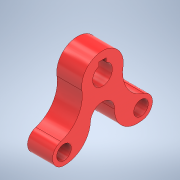
# Autodesk Inventor part: hw5
Saved by Autodesk Inventor 2021 (Build 250183000, 183)
## iProperties
Created: 2022-04-30
Part Number: hw5
Material: Generic
Document SubType Name: Modeling
Designer: authe
Density: 1 g/cm^3
Appearance: Light Red
Author: authe
Autodesk Inventor part; units mm, degrees
ref_plane "YZ Plane" through (0, 0, 0) normal (1, 0, 0) x (0, 1, 0)
ref_plane "XZ Plane" through (0, 0, 0) normal (0, 1, 0) x (-1, 0, 0)
ref_plane "XY Plane" through (0, 0, 0) normal (0, 0, 1) x (1, 0, 0)
sketch "Sketch1" plane through (0, 0, 0) normal (1, 0, 0) x (0, 1, 0)
  point P0 (0, 0)
sketch "Sketch2" plane through (0, 0, 0) normal (1, 0, 0) x (0, 1, 0)
  point P0 (0, 0)
sketch "Sketch3" plane through (0, 0, 0) normal (1, 0, 0) x (0, 1, 0)
  arc A0 (44.1588, 17.5) -> (44.1588, -17.5) centre (0, 0) ccw
  circle A1 centre (0, 0) radius 100
  line L0 (47.5, 0) -> (47.5, 17.5)
  line L1 (47.5, 17.5) -> (47.5, -17.5)
  line L2 (47.5, -17.5) -> (98.4568, -17.5)
  line L3 (47.5, 17.5) -> (98.4568, 17.5)
  line L4 (47.5, -17.5) -> (44.1588, -17.5)
  line L5 (47.5, 17.5) -> (44.1588, 17.5)
  line L6 (0, 0) -> (-170, 0)
  line L7 (-170, 0) -> (-230, 0)
  line L8 (-230, 0) -> (-230, 185)
  line L9 (-230, 185) -> (-230, -185)
  circle A2 centre (-230, -185) radius 35
  circle A3 centre (-230, -185) radius 55
  circle A4 centre (-230, 185) radius 35
  circle A5 centre (-230, 185) radius 55
  line L10 (-285, -185) -> (-284.7373, -179.631)
  arc A6 (-177.2131, 200.445) -> (-15.9759, 98.7156) centre (-38.9849, 240.8894) ccw
  arc A7 (-16.4956, -98.6301) -> (-177.1144, -200.1035) centre (-40.0152, -239.2575) ccw
  line L11 (-195.8559, -228.1182) -> (-204.1737, -233.5593)
  arc A8 (-172.1856, -58.1322) -> (-166.9431, 58.0929) centre (-170, 0) ccw
  arc A9 (-230, 15.6205) -> (-230, -15.6205) centre (-170, 0) ccw
  arc A10 (-285, 185) -> (-166.9431, 58.0929) centre (-160.3941, 182.5506) ccw
  arc A11 (-172.1856, -58.1322) -> (-285, -185) centre (-176.3183, -168.05) ccw
  line L12 (-47.5, 0) -> (62.5, 0)
  line L13 (62.5, 0) -> (62.5, 17.5)
  line L14 (62.5, 0) -> (62.5, -17.5)
  point P0 (-230, -84.1377)
  point P1 (-177.1744, 200.312)
  point P2 (-195.8559, -228.1182)
  point P3 (-177.1144, -200.1035)
  point P4 (-16.4956, -98.6301)
  point P5 (-4.7866, -99.8854)
  point P6 (-8.3439, 99.6513)
  point P7 (-15.9759, 98.7156)
  dimension "d0" = 95
  dimension "d1" = 200
  dimension "d2" = 17.5
  dimension "d3" = 35
  dimension "d4" = 170
  dimension "d6" = 60
  dimension "d7" = 185
  dimension "d8" = 370
  dimension "d9" = 70
  dimension "d10" = 110
  dimension "d11" = 70
  dimension "d12" = 110
  dimension "d17" = 110
  constraints: 30 end point, 26 point on circle, 12 centre point, 12 point on line, 7 coincident, 7 tangent, 2 horizontal, 2 perpendicular, 2 vertical, 1 midpoint, 1 parallel
  measures "d0" diameter of A0
  measures "d1" diameter of A1
  measures "d2" distance of L0.start L0.end
  measures "d3" distance of L0.end L1.end
  measures "d4" distance of L6.start L6.end
  measures "d6" distance of L7.start L7.end
  measures "d7" distance of L7.end L8.end
  measures "d8" distance of L8.end L9.end
  measures "d9" diameter of A2
  measures "d10" diameter of A3
  measures "d11" diameter of A4
  measures "d12" diameter of A5
  measures "d17" distance of L12.start L12.end
extrude "Extrusion1" add sketch "Sketch3" along normal blind 110 and the other way blind 10 contours A0 L6 A1 L3 L5 | A0 L4 L2 A1 L6 | L6 A8 A10 L8 A5 A6 A1 | A1 A7 A3 L9 A11 A8 L6 | L3 A1 L2 L14 L13 | A5 | A3 L11 L10 | A5 L8 A10 | L9 A3 A11
equation "\"d13\" = d10"
body "Solid1"
